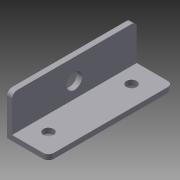
# Autodesk Inventor part: WheelBlockMount
Saved by Autodesk Inventor 2012 (Build 160160000, 160)
## iProperties
Created: 2012-01-07
Part Number: WheelBlockMount
Material: Aluminum-6061
Document SubType Name: Modeling
Designer: JesseK
Mass: 40.9458 g
Surface Area: 105.429 cm^2
Volume: 15.1092 cm^3
Density: 2.71 g/cm^3
Author: JesseK
Autodesk Inventor part; units mm, degrees
ref_plane "YZ Plane" through (0, 0, 0) normal (1, 0, 0) x (0, 1, 0)
ref_plane "XZ Plane" through (0, 0, 0) normal (0, 1, 0) x (-1, 0, 0)
ref_plane "XY Plane" through (0, 0, 0) normal (0, 0, 1) x (1, 0, 0)
sketch "Sketch1" plane through (0, 0, 0) normal (0, 0, 1) x (1, 0, 0)
  line L0 (0, 25.4) -> (0, 0)
  line L1 (0, 0) -> (25.4, 0)
  line L2 (25.4, 0) -> (25.4, 3.175)
  line L3 (25.4, 3.175) -> (3.175, 3.175)
  line L4 (3.175, 3.175) -> (3.175, 25.4)
  line L5 (3.175, 25.4) -> (0, 25.4)
  dimension "d0" = 3.175
  dimension "d1" = 3.175
  dimension "d2" = 25.4
  dimension "d3" = 25.4
  constraints: 12 end point, 4 parallel, 1 perpendicular, 1 vertical
  measures "d0" distance of L4.end L0.start
  measures "d1" distance of L1.end L2.end
  measures "d2" distance of L0.end L1.end
  measures "d3" distance of L0.start L0.end
extrude "Extrusion1" add sketch "Sketch1" along normal blind 76.2
fillet "Fillet1" radius 3.175 4 edges at (1.5875, 25.4, 76.2) (1.5875, 25.4, 0) (25.4, 1.5875, 0) (25.4, 1.5875, 76.2)
sketch "Sketch2" plane through (0, 0, 0) normal (-1, 0, 0) x (0, 0, 1)
  line L0 (0, 0) -> (76.2, 0) projected
  line L1 (3.175, 25.4) -> (73.025, 25.4) projected
  circle A0 centre (38.1, 12.7) radius 4.7625
  line L2 (38.1, 25.4) -> (38.1, 12.7)
  line L3 (38.1, 12.7) -> (38.1, 0)
  dimension "d7" = 9.525
  constraints: 4 end point, 2 midpoint, 1 centre point, 1 collinear, 1 perpendicular
  measures "d7" diameter of A0
extrude "Extrusion2" cut sketch "Sketch2" against normal up to next
sketch "Sketch3" plane through (0, 0, 0) normal (0, -1, 0) x (1, 0, 0)
  line L0 (22.225, 76.2) -> (0, 76.2) projected
  line L1 (0, 0) -> (0, 76.2) projected
  line L2 (22.225, 0) -> (0, 0) projected
  line L3 (25.4, 3.175) -> (25.4, 73.025) projected
  line L4 (0, 63.5) -> (12.7, 63.5)
  line L5 (12.7, 63.5) -> (25.4, 63.5)
  line L6 (12.7, 76.2) -> (12.7, 63.5)
  line L7 (12.7, 63.5) -> (12.7, 12.7)
  line L8 (12.7, 12.7) -> (12.7, 0)
  circle A0 centre (12.7, 63.5) radius 3.175
  circle A1 centre (12.7, 12.7) radius 3.175
  dimension "d10" = 12.7
  dimension "d11" = 6.35
  dimension "d12" = 6.35
  constraints: 10 end point, 4 point on line, 3 collinear, 3 perpendicular, 2 centre point, 2 coincident, 1 vertical
  measures "d10" distance of L6.start L4.end
  measures "d11" diameter of A0
  measures "d12" diameter of A1
extrude "Extrusion3" cut sketch "Sketch3" against normal up to next contours A0 L5 L6 | L6 L4 A0 | L7 A0 L4 | L5 A0 L7 | A1 L8 L7 | L7 L8 A1
body "Solid1"
